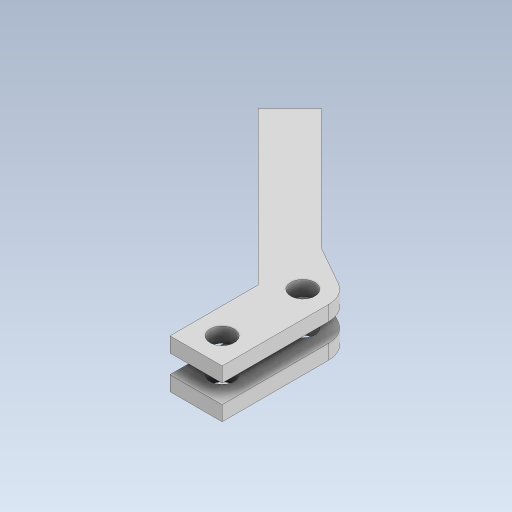
# Autodesk Inventor part: R2
Saved by Autodesk Inventor 2023 (Build 270158000, 158)
## iProperties
Created: 2022-09-16
Part Number: R2
Material: Generic
Document SubType Name: Modeling
Designer: Dave
Density: 1 g/cm^3
Appearance: Default
Author: Dave
## iProperties of the stored document R2_3DPrint.ipt
Created: 2022-09-16
Part Number: R2_3DPrint
Material: Generic
Document SubType Name: Modeling
Designer: Dave
Density: 1 g/cm^3
Appearance: Default
Author: Dave
Autodesk Inventor part; units mm, degrees
ref_plane "YZ Plane" through (0, 0, 0) normal (1, 0, 0) x (0, 1, 0)
ref_plane "XZ Plane" through (0, 0, 0) normal (0, 1, 0) x (-1, 0, 0)
ref_plane "XY Plane" through (0, 0, 0) normal (0, 0, 1) x (1, 0, 0)
sketch "Sketch1" plane through (0, 0, 0) normal (0, 1, 0) x (-1, 0, 0)
  line L0 (14, 0) -> (0, 0)
  line L1 (0, 0) -> (0, -35.7)
  line L2 (0, -35.7) -> (14, -35.7)
  line L3 (14, -35.7) -> (14, 0)
  circle A0 centre (7, -7) radius 3.25
  circle A1 centre (7, -28.7) radius 3.25
  arc A2 (14, -7) -> (0, -7) centre (7, -7) ccw
  line L4 (14, -35.7) -> (14, -40.7)
  line L5 (14, -40.7) -> (8.75, -40.7)
  line L6 (5.25, -40.7) -> (0, -40.7)
  line L7 (0, -40.7) -> (0, -35.7)
  line L8 (8.75, -40.7) -> (5.25, -40.7)
  line L9 (14, -40.7) -> (46.5741, -73.2741)
  line L10 (46.5741, -73.2741) -> (55.0594, -64.7888)
  line L11 (55.0594, -64.7888) -> (14, -23.7294)
  circle A3 centre (7, -28.7) radius 7
  line L12 (14, -40.7) -> (3.5544, -34.7933)
  point P0 (7, -35.7)
  point P1 (11.375, -40.7)
  point P2 (7, 0)
  point P3 (0, -28.7)
  dimension "d0" = 6.5
  dimension "d1" = 21.7
  dimension "d2" = 7
  dimension "d3" = 7
  dimension "d4" = 14
  dimension "d9" = 5
  dimension "d20" = 12
  dimension "d21" = 135
  constraints: 26 end point, 5 point on line, 4 coincident, 4 perpendicular, 3 centre point, 3 parallel, 2 horizontal, 2 midpoint, 2 point on circle, 2 vertical, 2 vertical alignment, 1 equal radius, 1 tangent, 4 other
  measures "d0" diameter of A0
  measures "d1" distance of A1.centre A0.centre
  measures "d2" distance from line of L0 A0.centre
  measures "d3" distance from line of L2 A1.centre
  measures "d4" distance of L1.end L2.end
  measures "d9" distance from line of L2 point (11.375, -40.7)
  measures "d20" distance of L9.end L10.end
  measures "d21" angle of L9 L4
extrude "Extrusion1" add sketch "Sketch1" along normal blind 4 contours L3 A2 L0 | A2 L1 L0 | A2 L3 A3 L1 | L11 L10 L9 L4 L3 | A3 | L3 L2 A3 | A3 L2 L12 | L4 L12 L2
fillet "Fillet1" radius 5 1 edges at (-14, 2, -40.7)
sketch "Sketch3" plane through (0, 4, 0) normal (0, 1, 0) x (1, 0, 0)
  line L0 (-14, 0) -> (0, 0) projected
  line L1 (0, 0) -> (0, 28.7) projected
  arc A0 (0, 28.7) -> (-3.5544, 34.7933) centre (-7, 28.7) ccw projected
  line L2 (-3.5544, 34.7933) -> (-13.4072, 40.3648) projected
  arc A1 (-14.4816, 41.1816) -> (-13.4072, 40.3648) centre (-10.946, 44.7171) ccw projected
  line L3 (-14.4816, 41.1816) -> (-46.5741, 73.2741) projected
  line L4 (-46.5741, 73.2741) -> (-55.0594, 64.7888) projected
  line L5 (-55.0594, 64.7888) -> (-14, 23.7294) projected
  line L6 (-14, 23.7294) -> (-14, 0) projected
  circle A2 centre (-7, 7) radius 3.25 projected
  circle A3 centre (-7, 28.7) radius 3.25 projected
  circle A4 centre (-7, 28.7) radius 7
  line L7 (-14, 23.7294) -> (-9.3072, 22.0912)
  line L8 (-14, 23.7294) -> (-14, 28.7)
  arc A5 (-12.6093, 32.8875) -> (-14.4816, 41.1816) centre (-17.092, 36.234) ccw
  line L9 (-14.4816, 41.1816) -> (-21.444, 48.144)
  point P0 (-3.5544, 34.7933)
  point P1 (-13.189, 40.2414)
  constraints: 6 end point, 6 point on circle, 2 centre point, 2 tangent, 1 coincident, 1 point on line, 1 vertical
extrude "Extrusion4" add sketch "Sketch3" along normal blind 2.5 contours L5 L4 L3 A1 L2 A5 A4 L8
mirror "Mirror3" about plane through (-33.2787, 6.5, -48.5018) normal (0, 1, 0) of "Extrusion4", "Fillet1", "Extrusion1"
body "Solid1"
